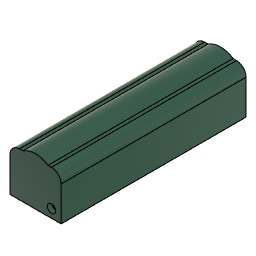
18650 Li-Ion Akku v2 (Autodesk Fusion 360 design; units mm, degrees)
Autodesk Fusion 360 part; units mm, degrees
sketch "Skizze1" plane through (0, 0, 0) normal (0, 0, 1) x (1, 0, 0)
  line L0 (0, 0) -> (21.3, 0)
  line L1 (21.3, 0) -> (21.3, 77)
  line L2 (21.3, 77) -> (0, 77)
  line L3 (0, 77) -> (0, 0)
  dimension "d1" = 21.3
  dimension "d2" = 77
  constraint horizontal L0
  constraint vertical L1
  constraint horizontal L2
  constraint vertical L3
  constraint coincident L0.start L3.end
  measures "d1" distance of L0.start L0.end
  measures "d2" distance of L0.start L2.end
extrude "Extrusion1" add sketch "Skizze1" along normal blind 18.4
fillet "Abrundung1" radius 4 2 edges at (21.3, 38.5, 18.4) (0, 38.5, 18.4)
sketch "Skizze3" plane through (0, 0, 0) normal (0, -1, 0) x (1, 0, 0)
  arc A0 (4, 18.4) -> (0, 14.4) centre (4, 14.4) ccw
  line L0 (0, 14.4) -> (0, 0)
  line L1 (0, 0) -> (21.3, 0)
  line L2 (21.3, 0) -> (21.3, 14.4)
  arc A1 (21.3, 14.4) -> (17.3, 18.4) centre (17.3, 14.4) ccw
  line L3 (17.3, 18.4) -> (4, 18.4)
  circle A2 centre (10.65, 10.75) radius 9.25
  dimension "d10" = 18.5
  dimension "d11" = 10.75
  dimension "d12" = 10.65
  measures "d10" diameter of A2
  measures "d11" distance of L1 A2.centre
  measures "d12" distance of L0 A2.centre
extrude "Extrusion3" add sketch "Skizze3" against normal blind 77 contours L3 A2 picked at (9.7432, 18.797)
sketch "Skizze4" plane through (0, 0, 0) normal (0, -1, 0) x (1, 0, 0)
  arc A0 (4, 18.4) -> (0, 14.4) centre (4, 14.4) ccw
  line L0 (0, 14.4) -> (0, 0)
  line L1 (0, 0) -> (21.3, 0)
  line L2 (21.3, 0) -> (21.3, 14.4)
  arc A1 (21.3, 14.4) -> (17.3, 18.4) centre (17.3, 14.4) ccw
  line L3 (17.3, 18.4) -> (15.85, 18.4)
  arc A2 (15.85, 18.4) -> (5.45, 18.4) centre (10.65, 10.75) ccw
  line L4 (5.45, 18.4) -> (4, 18.4)
  circle A3 centre (17.3, 3.5) radius 1.75
  dimension "d15" = 3.5
  dimension "d16" = 4
  dimension "d17" = 3.5
  measures "d15" diameter of A3
  measures "d16" distance of L2 A3.centre
  measures "d17" distance of L1 A3.centre
extrude "Extrusion4" cut sketch "Skizze4" against normal blind 2 contours A3
sketch "Skizze5" plane through (0, 77, 0) normal (0, 1, 0) x (-1, 0, 0)
  arc A0 (0, 14.4) -> (-4, 18.4) centre (-4, 14.4) ccw
  line L0 (-4, 18.4) -> (-5.45, 18.4)
  arc A1 (-5.45, 18.4) -> (-15.85, 18.4) centre (-10.65, 10.75) ccw
  line L1 (-15.85, 18.4) -> (-17.3, 18.4)
  arc A2 (-17.3, 18.4) -> (-21.3, 14.4) centre (-17.3, 14.4) ccw
  line L2 (-21.3, 14.4) -> (-21.3, 0)
  line L3 (-21.3, 0) -> (0, 0)
  line L4 (0, 0) -> (0, 14.4)
  circle A3 centre (-4, 3.5) radius 1.75
  dimension "d20" = 3.5
  dimension "d21" = 4
  dimension "d22" = 3.5
  measures "d20" diameter of A3
  measures "d21" distance of L4 A3.centre
  measures "d22" distance of L3 A3.centre
extrude "Extrusion5" cut sketch "Skizze5" against normal blind 2 contours A3
